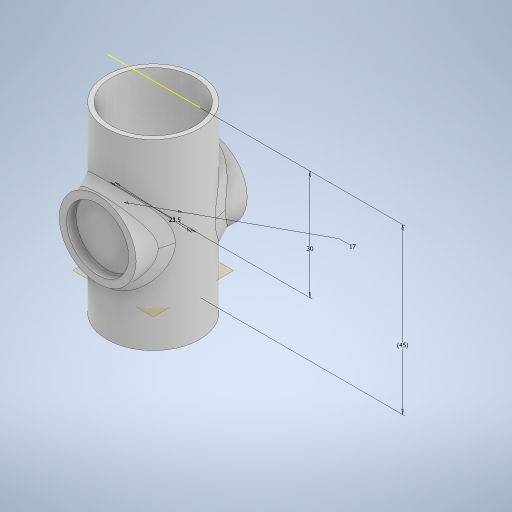
# Autodesk Inventor part: container
Saved by Autodesk Inventor 2024.2 (Build 282272000, 272)
## iProperties
Created: 2024-03-15
Part Number: container
Material: Generic
Document SubType Name: Sheet Metal
Designer: ellix
Density: 1 g/cm^3
Sheet Metal Rule: Default_mm
Appearance: Default
Author: ellix
Autodesk Inventor part; units mm, degrees
ref_plane "YZ Plane" through (0, 0, 0) normal (1, 0, 0) x (0, 1, 0)
ref_plane "XZ Plane" through (0, 0, 0) normal (0, 1, 0) x (-1, 0, 0)
ref_plane "XY Plane" through (0, 0, 0) normal (0, 0, 1) x (1, 0, 0)
sketch "Sketch1" plane through (0, 0, 0) normal (0, 1, 0) x (-1, 0, 0)
  circle A0 centre (0, 0) radius 11.45
  circle A1 centre (0, 0) radius 12.7
  dimension "d0" = 22.9
  dimension "d1" = 25.4
  constraints: 2 centre point, 2 coincident
  measures "d0" diameter of A0
  measures "d1" diameter of A1
extrude "Extrusion1" add sketch "Sketch1" along normal blind 45
sketch "Sketch2" plane through (0, 0, 0) normal (0, 0, 1) x (1, 0, 0)
  line L0 (12.7, 45) -> (-12.7, 45) projected
  line L1 (12.7, 0) -> (-12.7, 0) projected
  circle A0 centre (0, 15) radius 8.5
  circle A1 centre (0, 15) radius 10.5
  circle A2 centre (0, 15) radius 11.75
  point P0 (0, 0)
  point P1 (-1.1573, 60)
  point P2 (1.1573, 60)
  dimension "d4" = 17
  dimension "d5" = 21
  dimension "d10" = 23.5
  dimension "d15" = 30
  dimension "d16" = 45
  constraints: 3 centre point, 2 coincident
  measures "d4" diameter of A0
  measures "d5" diameter of A1
  measures "d10" diameter of A2
  measures "d15" distance from line of A2.centre L0
  measures "d16" distance between parallel lines of L1 L0
extrude "Extrusion2" add sketch "Sketch2" along normal mid plane 30.4 contours A0 | A1
sketch "Sketch3" plane through (0, 0, 0) normal (0, 1, 0) x (-1, 0, 0)
  point P0 (0, 0)
sketch "Sketch6" plane through (0, 0, 0) normal (0, 1, 0) x (-1, 0, 0)
  circle A0 centre (0, 0) radius 11.45 projected
sketch "Sketch7" plane through (0, 0, 0) normal (0, -1, 0) x (1, 0, 0)
  circle A0 centre (0, 0) radius 12.7 projected
  circle A1 centre (0, 0) radius 12.7 projected
  circle A2 centre (0, 0) radius 11.45 projected
sketch "Sketch9" plane through (0, 0, 0) normal (0, 1, 0) x (-1, 0, 0)
  circle A0 centre (0, 0) radius 12.7 projected
  line L0 (0, -12.7) -> (0, -28.75)
  line L1 (10.5, -28.75) -> (-10.5, -28.75) projected
  constraints: 2 end point, 1 midpoint, 1 vertical alignment, 1 other
ref_plane "Work Plane3" through (0, 0, 0) normal (0, 1, 0) x (1, 0, 0)
sketch "Sketch11" plane through (0, 0, 0) normal (0, 1, 0) x (1, 0, 0)
  circle A0 centre (0, 0) radius 11.45 projected
extrude "Extrusion11" cut sketch "Sketch11" along normal blind 85.25
chamfer "Chamfer1" distance 2 angle 45 2 edges at (-10.4996, 15.0897, -7.1448) (-10.4996, 15.0897, 7.1448)
sketch "Sketch12" plane through (0, 15, 15.2) normal (0, 0, 1) x (1, 0, 0)
  circle A0 centre (0, 0) radius 8.5 projected
  point P0 (0, -15)
extrude "Extrusion12" cut sketch "Sketch12" against normal blind 2.5
sketch "Sketch13" plane through (0, 15, -15.2) normal (0, 0, -1) x (-1, 0, 0)
  circle A0 centre (0, 0) radius 8.5 projected
  point P0 (0, -15)
extrude "Extrusion13" cut sketch "Sketch13" against normal blind 2.5
extrude "Extrusion14" add sketch "Sketch7" along normal blind 10
sketch "Sketch14" plane through (0, -10, 0) normal (0, -1, 0) x (1, 0, 0)
  circle A0 centre (0, 0) radius 12.7 projected
extrude "Extrusion15" add sketch "Sketch14" against normal blind 2
sketch "Sketch15" plane through (0, 45, 0) normal (0, 1, 0) x (1, 0, 0)
  circle A0 centre (0, 0) radius 12.7 projected
extrude "Extrusion16" cut sketch "Sketch15" against normal blind 5
equation "\"BendRadius\" = Thickness"
equation "\"BendReliefWidth\" = Thickness"
equation "\"BendReliefDepth\" = 0.5 * Thickness"
equation "\"CornerReliefSize\" = 4 * Thickness"
equation "\"MinimumRemnant\" = 2 * Thickness"
equation "\"TransitionRadius\" = BendRadius"
equation "\"JacobiRadiusSize\" = BendRadius"
equation "\"GapSize\" = Thickness"
equation "\"Thickness\" = 0.5"
body "Solid1"
